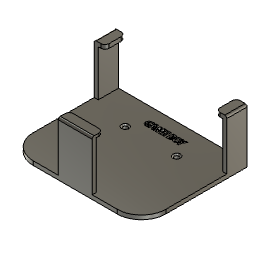
Nintendo Game Boy (Autodesk Fusion 360 design; units mm, degrees)
Autodesk Fusion 360 part; units mm, degrees
sketch "Sketch1" plane through (0, 0, 0) normal (0, 0, 1) x (1, 0, 0)
  line L0 (0, 0) -> (98, 0)
  line L1 (98, 0) -> (98, 78)
  line L2 (98, 78) -> (0, 78)
  line L3 (0, 78) -> (0, 0)
  dimension "d1" = 98
  dimension "d2" = 78
  constraint horizontal L0
  constraint vertical L1
  constraint horizontal L2
  constraint vertical L3
  constraint coincident L0.start L3.end
  measures "d1" distance of L0.start L0.end
  measures "d2" distance of L0.start L2.end
extrude "Extrude1" add sketch "Sketch1" along normal blind 40
sketch "Sketch2" plane through (0, 0, 40) normal (0, 0, 1) x (-1, 0, 0)
  line L0 (0, -78) -> (0, 0)
  line L1 (0, 0) -> (-98, 0)
  line L2 (-98, 0) -> (-98, -78)
  line L3 (-98, -78) -> (0, -78)
  line L4 (0, -78) -> (-8, -78)
  line L5 (-8, -78) -> (-8, -63)
  line L6 (-8, -63) -> (0, -63)
  line L7 (0, -63) -> (0, -78)
  line L8 (-98, -78) -> (-90, -78)
  line L9 (-90, -78) -> (-90, -63)
  line L10 (-90, -63) -> (-98, -63)
  line L11 (-98, -63) -> (-98, -78)
  line L12 (-49, 0) -> (-61.5, 0)
  line L13 (-61.5, 0) -> (-61.5, -8)
  line L14 (-61.5, -8) -> (-49, -8)
  line L15 (-49, -8) -> (-49, 0)
  line L16 (-49, 0) -> (-36.5, 0)
  line L17 (-36.5, 0) -> (-36.5, -8)
  line L18 (-36.5, -8) -> (-49, -8)
  line L19 (-49, -8) -> (-49, 0)
  dimension "d5" = 8
  dimension "d6" = 15
  dimension "d7" = 15
  dimension "d8" = 12.5
  dimension "d9" = 8
  dimension "d10" = 12.5
  dimension "d11" = 8
  constraint horizontal L4
  constraint vertical L5
  constraint horizontal L6
  constraint vertical L7
  constraint coincident L0.start L3.end
  constraint horizontal L8
  constraint vertical L9
  constraint horizontal L10
  constraint vertical L11
  constraint coincident L2.end L3.start
  constraint horizontal L12
  constraint vertical L13
  constraint horizontal L14
  constraint vertical L15
  constraint midpoint L1 L12.start
  constraint horizontal L16
  constraint vertical L17
  constraint horizontal L18
  constraint vertical L19
  measures "d5" distance of L0.start L4.end
  measures "d6" distance of L0.start L6.end
  measures "d7" distance of L2.end L10.end
  measures "d8" distance of L12.start L12.end
  measures "d9" distance of L12.start L14.end
  measures "d10" distance of L12.start L16.end
  measures "d11" distance of L12.start L14.end
extrude "Extrude2" cut sketch "Sketch2" against normal blind 37 contours L0 L1 L2 L3 L5 L6 L9 L10 L13 L14 L17 L18
sketch "Sketch3" plane through (0, 63, 0) normal (0, -1, 0) x (1, 0, 0)
  line L0 (8, 40) -> (0, 40)
  line L1 (0, 40) -> (0, 3)
  line L2 (0, 3) -> (8, 3)
  line L3 (8, 3) -> (8, 40)
  line L4 (8, 3) -> (3, 3)
  line L5 (3, 3) -> (3, 37)
  line L6 (3, 37) -> (8, 37)
  line L7 (8, 37) -> (8, 3)
  dimension "d14" = 5
  constraint horizontal L4
  constraint vertical L5
  constraint horizontal L6
  constraint vertical L7
  constraint coincident L2.end L3.start
  measures "d14" distance of L2.end L4.end
extrude "Extrude3" cut sketch "Sketch3" against normal blind 15 contours L2 L3 L4 L5 L6 L7
sketch "Sketch4" plane through (0, 63, 0) normal (0, -1, 0) x (1, 0, 0)
  line L0 (98, 40) -> (90, 40)
  line L1 (90, 40) -> (90, 3)
  line L2 (90, 3) -> (98, 3)
  line L3 (98, 3) -> (98, 40)
  line L4 (90, 3) -> (95, 3)
  line L5 (95, 3) -> (95, 37)
  line L6 (95, 37) -> (90, 37)
  line L7 (90, 37) -> (90, 3)
  dimension "d17" = 5
  dimension "d18" = 34
  constraint horizontal L4
  constraint vertical L5
  constraint horizontal L6
  constraint vertical L7
  constraint coincident L1.end L2.start
  measures "d17" distance of L1.end L4.end
  measures "d18" distance of L1.end L6.end
extrude "Extrude4" cut sketch "Sketch4" against normal blind 15 contours L1 L2 L4 L5 L6 L7
sketch "Sketch5" plane through (61.5, 0, 0) normal (1, 0, 0) x (0, 1, 0)
  line L0 (8, 40) -> (0, 40)
  line L1 (0, 40) -> (0, 3)
  line L2 (0, 3) -> (8, 3)
  line L3 (8, 3) -> (8, 40)
  line L4 (8, 3) -> (3, 3)
  line L5 (3, 3) -> (3, 38)
  line L6 (3, 38) -> (8, 38)
  line L7 (8, 38) -> (8, 3)
  dimension "d21" = 5
  dimension "d22" = 35
  constraint horizontal L4
  constraint vertical L5
  constraint horizontal L6
  constraint vertical L7
  constraint coincident L2.end L3.start
  measures "d21" distance of L2.end L4.end
  measures "d22" distance of L2.end L6.end
extrude "Extrude5" cut sketch "Sketch5" against normal blind 25 contours L2 L3 L4 L5 L6 L7
fillet "Fillet1" radius 18 1 edges at (98, 0, 1.5)
fillet "Fillet2" radius 18 1 edges at (0, 0, 1.5)
sketch "Logo" plane through (0, 0, 3) normal (0, 0, 1) x (1, 0, 0)
  line L0 (61.6174, 66.2149) -> (61.3315, 64.0782)
  line L1 (61.3315, 64.0782) -> (60.2029, 64.0782)
  line L2 (61.2261, 67.5691) -> (62.129, 68.9534)
  line L3 (59.4054, 68.9534) -> (60.6242, 68.9534)
  line L4 (62.129, 68.9534) -> (63.3779, 68.9534)
  line L5 (60.5339, 66.5158) -> (59.4054, 68.9534)
  line L6 (60.2029, 64.0782) -> (60.5339, 66.5158)
  line L7 (60.6242, 68.9534) -> (61.2261, 67.5691)
  line L8 (63.3779, 68.9534) -> (61.6174, 66.2149)
  line L9 (51.1293, 68.9534) -> (48.2854, 68.9534)
  line L10 (49.2484, 67.8701) -> (50.9638, 67.8701)
  line L11 (47.6083, 64.0782) -> (50.4371, 64.0782)
  line L12 (50.5876, 65.1616) -> (48.8723, 65.1616)
  line L13 (50.6177, 67.0876) -> (49.1431, 67.0876)
  line L14 (48.8723, 65.1616) -> (48.9776, 66.0042)
  line L15 (50.9638, 67.8701) -> (51.1293, 68.9534)
  line L16 (49.1431, 67.0876) -> (49.2484, 67.8701)
  line L17 (50.4672, 66.0042) -> (50.6177, 67.0876)
  line L18 (50.4371, 64.0782) -> (50.5876, 65.1616)
  line L19 (48.2854, 68.9534) -> (47.6083, 64.0782)
  line L20 (48.9776, 66.0042) -> (50.4672, 66.0042)
  line L21 (39.904, 65.5227) -> (40.9272, 65.5227)
  line L22 (40.9272, 65.5227) -> (41.1078, 64.0782)
  line L23 (41.1078, 64.0782) -> (42.9586, 64.0782)
  line L24 (42.9586, 64.0782) -> (43.8163, 66.7264)
  line L25 (43.8163, 66.7264) -> (44.2377, 64.0782)
  line L26 (44.2377, 64.0782) -> (45.2158, 64.0782)
  line L27 (45.2158, 64.0782) -> (46.2992, 66.8769)
  line L28 (46.2992, 66.8769) -> (46.4797, 64.0782)
  line L29 (46.4797, 64.0782) -> (47.5631, 64.0782)
  line L30 (47.5631, 64.0782) -> (47.2622, 68.9534)
  line L31 (47.2622, 68.9534) -> (45.9681, 68.9534)
  line L32 (45.9681, 68.9534) -> (44.96, 66.3804)
  line L33 (44.96, 66.3804) -> (44.5687, 68.9534)
  line L34 (44.5687, 68.9534) -> (43.4101, 68.9534)
  line L35 (43.4101, 68.9534) -> (42.0859, 64.9509)
  line L36 (42.0859, 64.9509) -> (41.5893, 68.9534)
  line L37 (41.5893, 68.9534) -> (40.1448, 68.9534)
  line L38 (40.1448, 68.9534) -> (38.5347, 64.9058)
  line L39 (38.5347, 64.9058) -> (38.7453, 66.4858)
  line L40 (38.7453, 66.4858) -> (36.7892, 66.4858)
  line L41 (36.7892, 66.4858) -> (36.6537, 65.5227)
  line L42 (36.6537, 65.5227) -> (37.5115, 65.5227)
  line L43 (37.5115, 65.5227) -> (37.4513, 65.1917)
  spline S0 degree 3 poles (37.4513, 65.1917) (37.3008, 65.1014) (36.9548, 65.0863) (36.8193, 65.0863) (36.6839, 65.0863) (35.6757, 65.1766) (35.7209, 66.26) (35.766, 67.3434) (37.2106, 68.3516) (38.9259, 67.7948) knots 23 23 23 23 24 24 24 25 25 25 26 26 26 26
  line L44 (38.9259, 67.7948) -> (39.0915, 68.8331)
  spline S1 degree 3 poles (39.0915, 68.8331) (37.9479, 69.2243) (34.9443, 69.0054) (34.6374, 66.3202) knots 27 27 27 27 28 28 28 28
  spline S2 degree 3 poles (34.6374, 66.3202) (34.4569, 64.7402) (35.9015, 63.9878) (36.8644, 64.0029) knots 28 28 28 28 29 29 29 29
  spline S3 degree 3 poles (36.8644, 64.0029) (37.4212, 63.9728) (38.0532, 64.1835) (38.2789, 64.3039) knots 29 29 29 29 30 30 30 30
  line L45 (38.2789, 64.3039) -> (38.2036, 64.0782)
  line L46 (38.2036, 64.0782) -> (39.3473, 64.0782)
  line L47 (39.3473, 64.0782) -> (39.904, 65.5227)
  line L48 (40.3103, 66.4858) -> (40.6865, 67.4939)
  line L49 (40.6865, 67.4939) -> (40.8069, 66.4858)
  line L50 (40.8069, 66.4858) -> (40.3103, 66.4858)
  spline S4 degree 3 poles (58.0661, 67.9603) (58.3822, 67.9603) (59.0593, 67.7497) (58.8937, 66.4858) knots 0 0 0 0 1 1 1 1
  spline S5 degree 3 poles (58.8937, 66.4858) (58.7283, 65.2218) (57.9458, 65.0713) (57.6599, 65.1014) knots 1 1 1 1 2 2 2 2
  spline S6 degree 3 poles (57.6599, 65.1014) (57.374, 65.1315) (56.7871, 65.3271) (56.9527, 66.4858) knots 2 2 2 2 3 3 3 3
  spline S7 degree 3 poles (56.9527, 66.4858) (57.1182, 67.6443) (57.7351, 67.9754) (58.0661, 67.9603) knots 3 3 3 3 4 4 4 4
  spline S8 degree 3 poles (58.1865, 68.9986) (57.404, 69.0287) (56.2755, 68.5773) (55.8994, 66.7565) knots 0 0 0 0 1 1 1 1
  spline S9 degree 3 poles (55.8994, 66.7565) (55.5232, 64.9359) (56.5314, 64.1986) (57.4642, 64.0782) knots 1 1 1 1 2 2 2 2
  spline S10 degree 3 poles (57.4642, 64.0782) (58.3972, 63.9578) (59.7063, 64.5446) (59.9471, 66.2901) knots 2 2 2 2 3 3 3 3
  spline S11 degree 3 poles (59.9471, 66.2901) (60.1878, 68.0356) (59.3301, 68.9534) (58.1865, 68.9986) knots 3 3 3 3 4 4 4 4
  line L51 (51.8968, 64.0782) -> (52.5739, 68.9534)
  line L52 (52.5739, 68.9534) -> (54.6504, 68.9534)
  spline S12 degree 3 poles (54.6504, 68.9534) (55.147, 68.9534) (55.8693, 68.3817) (55.779, 67.6143) knots 2 2 2 2 3 3 3 3
  spline S13 degree 3 poles (55.779, 67.6143) (55.6887, 66.8468) (55.4479, 66.8017) (55.2824, 66.6813) knots 3 3 3 3 4 4 4 4
  spline S14 degree 3 poles (55.2824, 66.6813) (55.5382, 66.4556) (55.794, 66.0945) (55.6887, 65.4174) knots 4 4 4 4 5 5 5 5
  spline S15 degree 3 poles (55.6887, 65.4174) (55.5833, 64.7402) (55.0266, 64.0782) (54.0485, 64.0782) knots 5 5 5 5 6 6 6 6
  line L53 (54.0485, 64.0782) -> (51.8968, 64.0782)
  line L54 (53.1607, 65.1616) -> (54.0184, 65.1616)
  spline S16 degree 3 poles (54.0184, 65.1616) (54.4849, 65.1616) (54.5902, 65.5227) (54.6053, 65.6431) knots 1 1 1 1 2 2 2 2
  spline S17 degree 3 poles (54.6053, 65.6431) (54.6203, 65.7635) (54.4849, 66.0042) (54.2442, 66.0042) knots 2 2 2 2 3 3 3 3
  line L55 (54.2442, 66.0042) -> (53.2811, 66.0042)
  line L56 (53.2811, 66.0042) -> (53.1607, 65.1616)
  line L57 (53.4316, 67.0876) -> (54.0636, 67.0876)
  spline S18 degree 3 poles (54.0636, 67.0876) (54.53, 67.0876) (54.6203, 67.3885) (54.6353, 67.5089) knots 1 1 1 1 2 2 2 2
  spline S19 degree 3 poles (54.6353, 67.5089) (54.6504, 67.6293) (54.515, 67.8701) (54.2742, 67.8701) knots 2 2 2 2 3 3 3 3
  line L58 (54.2742, 67.8701) -> (53.5369, 67.8701)
  line L59 (53.5369, 67.8701) -> (53.4316, 67.0876)
extrude "Extrude7" cut sketch "Logo" against normal blind 2
fillet "Fillet3" radius 3 6 edges at (8, 63, 38.5) (90, 63, 38.5) (61.5, 8, 39) (36.5, 8, 39) (90, 78, 38.5) (8, 78, 38.5)
fillet "Fillet4" radius 1.5 3 edges at (98, 70.5, 40) (49, 0, 40) (0, 70.5, 40)
hole "Hole3" at (30, 56, 3) direction (0, 0, -1) diameter 3.5 depth 3 tip angle 118 countersink diameter 5.5 countersink angle 90
hole "Hole4" at (68, 56, 3) direction (0, 0, -1) diameter 3.5 depth 3 tip angle 118 countersink diameter 5.5 countersink angle 90
sketch "game-boy-logo" plane through (0, 0, 0) normal (0, 0, 1) x (1, 0, 0)
  line L0 (63.3779, 65.9534) -> (61.6174, 63.2149)
  line L1 (61.3315, 61.0782) -> (60.2029, 61.0782)
  line L2 (60.5339, 63.5158) -> (59.4054, 65.9534)
  line L3 (60.2029, 61.0782) -> (60.5339, 63.5158)
  line L4 (62.129, 65.9534) -> (63.3779, 65.9534)
  line L5 (61.6174, 63.2149) -> (61.3315, 61.0782)
  line L6 (60.6242, 65.9534) -> (61.2261, 64.5691)
  line L7 (61.2261, 64.5691) -> (62.129, 65.9534)
  line L8 (59.4054, 65.9534) -> (60.6242, 65.9534)
  line L9 (49.2484, 64.8701) -> (50.9638, 64.8701)
  line L10 (50.9638, 64.8701) -> (51.1293, 65.9534)
  line L11 (50.6177, 64.0876) -> (49.1431, 64.0876)
  line L12 (47.6083, 61.0782) -> (50.4371, 61.0782)
  line L13 (49.1431, 64.0876) -> (49.2484, 64.8701)
  line L14 (51.1293, 65.9534) -> (48.2854, 65.9534)
  line L15 (48.8723, 62.1616) -> (48.9776, 63.0042)
  line L16 (48.2854, 65.9534) -> (47.6083, 61.0782)
  line L17 (48.9776, 63.0042) -> (50.4672, 63.0042)
  line L18 (50.5876, 62.1616) -> (48.8723, 62.1616)
  line L19 (50.4371, 61.0782) -> (50.5876, 62.1616)
  line L20 (50.4672, 63.0042) -> (50.6177, 64.0876)
  line L21 (39.904, 62.5227) -> (40.9272, 62.5227)
  line L22 (40.9272, 62.5227) -> (41.1078, 61.0782)
  line L23 (41.1078, 61.0782) -> (42.9586, 61.0782)
  line L24 (42.9586, 61.0782) -> (43.8163, 63.7264)
  line L25 (43.8163, 63.7264) -> (44.2377, 61.0782)
  line L26 (44.2377, 61.0782) -> (45.2158, 61.0782)
  line L27 (45.2158, 61.0782) -> (46.2992, 63.8769)
  line L28 (46.2992, 63.8769) -> (46.4797, 61.0782)
  line L29 (46.4797, 61.0782) -> (47.5631, 61.0782)
  line L30 (47.5631, 61.0782) -> (47.2622, 65.9534)
  line L31 (47.2622, 65.9534) -> (45.9681, 65.9534)
  line L32 (45.9681, 65.9534) -> (44.96, 63.3804)
  line L33 (44.96, 63.3804) -> (44.5687, 65.9534)
  line L34 (44.5687, 65.9534) -> (43.4101, 65.9534)
  line L35 (43.4101, 65.9534) -> (42.0859, 61.9509)
  line L36 (42.0859, 61.9509) -> (41.5893, 65.9534)
  line L37 (41.5893, 65.9534) -> (40.1448, 65.9534)
  line L38 (40.1448, 65.9534) -> (38.5347, 61.9058)
  line L39 (38.5347, 61.9058) -> (38.7453, 63.4858)
  line L40 (38.7453, 63.4858) -> (36.7892, 63.4858)
  line L41 (36.7892, 63.4858) -> (36.6537, 62.5227)
  line L42 (36.6537, 62.5227) -> (37.5115, 62.5227)
  line L43 (37.5115, 62.5227) -> (37.4513, 62.1917)
  spline S0 degree 3 poles (37.4513, 62.1917) (37.3008, 62.1014) (36.9548, 62.0863) (36.8193, 62.0863) (36.6839, 62.0863) (35.6757, 62.1766) (35.7209, 63.26) (35.766, 64.3434) (37.2106, 65.3516) (38.9259, 64.7948) knots 23 23 23 23 24 24 24 25 25 25 26 26 26 26
  line L44 (38.9259, 64.7948) -> (39.0915, 65.8331)
  spline S1 degree 3 poles (39.0915, 65.8331) (37.9479, 66.2243) (34.9443, 66.0054) (34.6374, 63.3202) knots 27 27 27 27 28 28 28 28
  spline S2 degree 3 poles (34.6374, 63.3202) (34.4569, 61.7402) (35.9015, 60.9878) (36.8644, 61.0029) knots 28 28 28 28 29 29 29 29
  spline S3 degree 3 poles (36.8644, 61.0029) (37.4212, 60.9728) (38.0532, 61.1835) (38.2789, 61.3039) knots 29 29 29 29 30 30 30 30
  line L45 (38.2789, 61.3039) -> (38.2036, 61.0782)
  line L46 (38.2036, 61.0782) -> (39.3473, 61.0782)
  line L47 (39.3473, 61.0782) -> (39.904, 62.5227)
  spline S4 degree 3 poles (58.1865, 65.9986) (57.404, 66.0287) (56.2755, 65.5773) (55.8994, 63.7565) knots 0 0 0 0 1 1 1 1
  spline S5 degree 3 poles (55.8994, 63.7565) (55.5232, 61.9359) (56.5314, 61.1986) (57.4642, 61.0782) knots 1 1 1 1 2 2 2 2
  spline S6 degree 3 poles (57.4642, 61.0782) (58.3972, 60.9578) (59.7063, 61.5446) (59.9471, 63.2901) knots 2 2 2 2 3 3 3 3
  spline S7 degree 3 poles (59.9471, 63.2901) (60.1878, 65.0356) (59.3301, 65.9534) (58.1865, 65.9986) knots 3 3 3 3 4 4 4 4
  line L48 (51.8968, 61.0782) -> (52.5739, 65.9534)
  line L49 (52.5739, 65.9534) -> (54.6504, 65.9534)
  spline S8 degree 3 poles (54.6504, 65.9534) (55.147, 65.9534) (55.8693, 65.3817) (55.779, 64.6143) knots 2 2 2 2 3 3 3 3
  spline S9 degree 3 poles (55.779, 64.6143) (55.6887, 63.8468) (55.4479, 63.8017) (55.2824, 63.6813) knots 3 3 3 3 4 4 4 4
  spline S10 degree 3 poles (55.2824, 63.6813) (55.5382, 63.4556) (55.794, 63.0945) (55.6887, 62.4174) knots 4 4 4 4 5 5 5 5
  spline S11 degree 3 poles (55.6887, 62.4174) (55.5833, 61.7402) (55.0266, 61.0782) (54.0485, 61.0782) knots 5 5 5 5 6 6 6 6
  line L50 (54.0485, 61.0782) -> (51.8968, 61.0782)
extrude "Extrude6" [rolled back] along distance 3 taper angle 0
hole "Hole1" [rolled back] hole depth 3 hole diameter 3.5 tip angle 118 csdiameter 5.5 csangle 90 ref dim1 22 ref dim2 30
hole "Hole2" [rolled back] hole depth 3 hole diameter 3.5 tip angle 118 csdiameter 5.5 csangle 90 ref dim1 22 ref dim2 30
